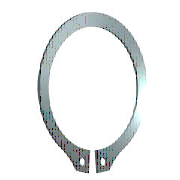
# Autodesk Inventor part: Кольцо стопорное наружное
Saved by Autodesk Inventor 2025 (Build 290162010, 162A)
## iProperties
IsCustomPart: 0
Created: 2023-01-19
Part Number: Кольцо стопорное наружное
Material: Steel, Mild
Description: American National Standard Metric Tapered Retaining Rings - Basic External Series - 3AMI
Document SubType Name: Modeling
Standard: ANSI B 27.7M
Designer: pokla
Standards Organization: ANSI
Language: en-US
Size Designation: 3AMI-17
Categories: <MemberInstance><Categories><Category DisplayName="Shaft Parts" InternalName="7f7aeb1f-a693-4053-b835-cee3144e0d98" Mnemonic="SHFT"><Category DisplayName="Circlips" InternalName="413b042a-1f46-4051-a560-0e0e417af91f" Mnemonic="CLIP"><CategoryParameter DisplayName="Thickness" InternalName="230c7f7c-2544-4c6d-b8d5-773e831b23fa" Mnemonic="thick"/><CategoryParameter DisplayName="Groove Diameter" InternalName="4054b45c-161d-4ad6-befb-f30b3855ce84" Mnemonic="grvdia"/><CategoryParameter DisplayName="Groove Width" InternalName="4dde6996-4bf1-443b-8317-d4f4fc6b9be0" Mnemonic="NB"/><CategoryParameter DisplayName="Shaft Diameter" InternalName="a433c9ab-b9eb-4798-a453-f2210a67728e" Mnemonic="shaftdia"/><Category DisplayName="External" InternalName="a9a2b132-a8be-48ab-9c3d-0c324a909558" Mnemonic="OUCLIP"><CategoryParameter DisplayName="Shaft Diameter Min." InternalName="62b77b9b-1e86-4b9a-9911-d7c0fa48fc9a" Mnemonic="shaftdiamin"/><CategoryParameter DisplayName="Outer Diameter" InternalName="a3599e7b-be7c-41b5-9a50-6dab253b0906" Mnemonic="outdia"/></Category></Category></Category><Category DisplayName="DataType" InternalName="23b78d0f-2648-40c6-8793-ca6db495c9e8" Mnemonic="DATATYPE"><CategoryParameter DisplayName="DisplayName" InternalName="05415f3d-3907-474b-a020-eb9d644f4cf3" Mnemonic="DISPLAYNAME"/><CategoryParameter DisplayName="Standard" InternalName="0c0a119c-1e12-4c84-803f-101930972f5e" Mnemonic="STANDARD"/><CategoryParameter DisplayName="Description" InternalName="13903e3d-64b1-4950-80da-f627842ea37f" Mnemonic="DESCRIPTION"/><CategoryParameter DisplayName="Designation" InternalName="2675968c-4ce5-49e0-a4f5-552d29089031" Mnemonic="DESIGNATION"/><CategoryParameter DisplayName="Default Row" InternalName="2af9ec52-faaa-4026-b378-f9fa4afca842" Mnemonic="DEFAULTROW"/><CategoryParameter DisplayName="Folder Name" InternalName="3f06958e-8713-4116-9be7-ed6184ecc97b" Mnemonic="FOLDERNAME"/><CategoryParameter DisplayName="Revision Guid" InternalName="45a75005-10b1-4dfc-8d6d-dfe629f0b93c" Mnemonic="REVISIONGUID"/><CategoryParameter DisplayName="FileName" InternalName="8b46a4cc-9585-4fed-90c3-899f57e09a73" Mnemonic="FILENAME"/><CategoryParameter DisplayName="StdsOrg" InternalName="8f5914e1-4693-403f-8ab5-d37768198c9d" Mnemonic="STDSORG"/><CategoryParameter DisplayName="Family Version" InternalName="914462f6-6e19-4b14-ba84-155b9680b1d0" Mnemonic="FAMILYREVISION"/><CategoryParameter DisplayName="Standard Revision" InternalName="91d5a463-65c2-4fde-b823-3b7fea5e8e17" Mnemonic="STANDARDREVISION"/><CategoryParameter DisplayName="Member Revision" InternalName="a65d44b9-392f-4f4f-857b-e4b3d54996fe" Mnemonic="MEMBERREVISION"/><CategoryParameter DisplayName="ClipFormat" InternalName="bc51e27b-3422-4e78-93ef-cec197ddf230" Mnemonic="CLIPFORMAT"/><CategoryParameter DisplayName="Manufacturer" InternalName="cd6c7a72-a28a-4e50-99a9-2c7f4e13e5ad" Mnemonic="MANUFACTURER"/><CategoryParameter DisplayName="InternalName" InternalName="cf1d0246-76d9-4b4a-8305-fa0409afb5c1" Mnemonic="INTERNALNAME"/><CategoryParameter DisplayName="IsMetric" InternalName="e2385c5b-1ea4-4823-96a8-8de651266ec3" Mnemonic="ISMETRIC"/><Category DisplayName="Part" InternalName="c0e0b642-3bcb-4cc8-9e80-f96d35c4afa4" Mnemonic="PART"><CategoryParameter DisplayName="Part Number" InternalName="016b6077-bfbe-49bd-92c9-d8d59c39c941" Mnemonic="PARTNUMBER"/><CategoryParameter DisplayName="Stock Number" InternalName="4dba7c1c-e26c-444e-836c-b08b433409a8" Mnemonic="STOCKNUMBER"/><CategoryParameter DisplayName="Material Key" InternalName="5c9a8adb-dd2b-4535-b97f-0a94a95fe41f" Mnemonic="MATERIALKEY"/><CategoryParameter DisplayName="Material" InternalName="818a152a-d3c3-49ca-80ee-df7d91421b8e" Mnemonic="MATERIAL"/></Category></Category><Category DisplayName="Legacy Map DA" InternalName="924fff40-ddd0-4eff-ad42-30e3774ef79e" Mnemonic="LEGACYMAPDA"><CategoryParameter DisplayName="DACookie" InternalName="316934ee-8fe1-4c7a-9c36-f2d79e1add1a" Mnemonic="DACOOKIE"/></Category></Categories><FamilyTemplate Id="A2773e"><FamilyTemplateParameters><FamilyTemplateParameter ObjectType="kUserParameterObject" ValueType="xs:double" Id="3" ObjectReferenceKey="tt"/><FamilyTemplateParameter ObjectType="kUserParameterObject" ValueType="xs:double" Id="4" ObjectReferenceKey="g1"/><FamilyTemplateParameter ObjectType="kUserParameterObject" ValueType="xs:double" Id="8" ObjectReferenceKey="Diam5"/><FamilyTemplateParameter ObjectType="kUserParameterObject" ValueType="xs:double" Id="9" ObjectReferenceKey="b"/><FamilyTemplateParameter ObjectType="kUserParameterObject" ValueType="xs:double" Id="10" ObjectReferenceKey="ParA"/><FamilyTemplateParameter ObjectType="kUserParameterObject" ValueType="xs:string" Id="117" ObjectReferenceKey="TEMPLATE"/><FamilyTemplateParameter ObjectType="kPropertyObject" ValueType="xs:string" Id="100" ObjectReferenceKey="{32853F0F-3444-11d1-9E93-0060B03C1CA6}" SubObjectId="52"/><FamilyTemplateParameter ObjectType="kPropertyObject" ValueType="xs:string" Id="105" ObjectReferenceKey="{32853F0F-3444-11d1-9E93-0060B03C1CA6}" SubObjectId="5"/><FamilyTemplateParameter ObjectType="kPartComponentDefinitionObject" ValueType="xs:string" Id="110" SubObjectId="Material"/></FamilyTemplateParameters></FamilyTemplate><CategoryParameterMap><ParamToTemplateMap><ParamToTemplate CategoryParameter="//CategoryParameter[@InternalName='05415f3d-3907-474b-a020-eb9d644f4cf3']" ConstantValue="ANSI B 27.7M"/><ParamToTemplate CategoryParameter="//CategoryParameter[@InternalName='cf1d0246-76d9-4b4a-8305-fa0409afb5c1']" ConstantValue="84A47C50-19B2-4694-A97F-23806F30E450"/><ParamToTemplate CategoryParameter="//CategoryParameter[@InternalName='3f06958e-8713-4116-9be7-ed6184ecc97b']" ConstantValue="ANSI B 27.7M(2)"/><ParamToTemplate CategoryParameter="//CategoryParameter[@InternalName='914462f6-6e19-4b14-ba84-155b9680b1d0']" ConstantValue="10"/><ParamToTemplate CategoryParameter="//CategoryParameter[@InternalName='bc51e27b-3422-4e78-93ef-cec197ddf230']" ConstantValue="CF_INVENTOR.STDPARTS"/><ParamToTemplate CategoryParameter="//CategoryParameter[@InternalName='e2385c5b-1ea4-4823-96a8-8de651266ec3']" ConstantValue="true"/><ParamToTemplate CategoryParameter="//CategoryParameter[@InternalName='13903e3d-64b1-4950-80da-f627842ea37f']" ConstantValue="American National Standard Metric Tapered Retaining Rings - Basic External Series - 3AMI"/><ParamToTemplate CategoryParameter="//CategoryParameter[@InternalName='8f5914e1-4693-403f-8ab5-d37768198c9d']" ConstantValue="ANSI"/><ParamToTemplate CategoryParameter="//CategoryParameter[@InternalName='0c0a119c-1e12-4c84-803f-101930972f5e']" ConstantValue="ANSI B 27.7M"/><ParamToTemplate CategoryParameter="//CategoryParameter[@InternalName='cd6c7a72-a28a-4e50-99a9-2c7f4e13e5ad']" TemplateParameter="104"/><ParamToTemplate CategoryParameter="//CategoryParameter[@InternalName='91d5a463-65c2-4fde-b823-3b7fea5e8e17']" TemplateParameter="103"/><ParamToTemplate CategoryParameter="//CategoryParameter[@InternalName='45a75005-10b1-4dfc-8d6d-dfe629f0b93c']" ConstantValue="d6c6cd7d-6663-4866-9fff-0a208e8d6214"/><ParamToTemplate CategoryParameter="//CategoryParameter[@InternalName='2af9ec52-faaa-4026-b378-f9fa4afca842']" ConstantValue="10"/><ParamToTemplate CategoryParameter="//CategoryParameter[@InternalName='8b46a4cc-9585-4fed-90c3-899f57e09a73']" ConstantValue="ANSI B 27.7M - 3AMI-17"/><ParamToTemplate CategoryParameter="//CategoryParameter[@InternalName='a65d44b9-392f-4f4f-857b-e4b3d54996fe']" ConstantValue="E8632F14-C031-4BBE-B420-CE7F4CDB762D"/><ParamToTemplate CategoryParameter="//CategoryParameter[@InternalName='a433c9ab-b9eb-4798-a453-f2210a67728e']" ConstantValue="17"/><ParamToTemplate CategoryParameter="//CategoryParameter[@InternalName='230c7f7c-2544-4c6d-b8d5-773e831b23fa']" ConstantValue="0,9"/><ParamToTemplate CategoryParameter="//CategoryParameter[@InternalName='4054b45c-161d-4ad6-befb-f30b3855ce84']" ConstantValue="15,75"/><ParamToTemplate CategoryParameter="//CategoryParameter[@InternalName='4dde6996-4bf1-443b-8317-d4f4fc6b9be0']" ConstantValue="1"/><ParamToTemplate CategoryParameter="//CategoryParameter[@InternalName='316934ee-8fe1-4c7a-9c36-f2d79e1add1a']" ConstantValue="*ANS~A2773AMI~3AMI-17*"/><ParamToTemplate CategoryParameter="//CategoryParameter[@InternalName='2675968c-4ce5-49e0-a4f5-552d29089031']" TemplateParameter="100"/><ParamToTemplate CategoryParameter="//CategoryParameter[@InternalName='818a152a-d3c3-49ca-80ee-df7d91421b8e']" TemplateParameter="110"/><ParamToTemplate CategoryParameter="//CategoryParameter[@InternalName='016b6077-bfbe-49bd-92c9-d8d59c39c941']" TemplateParameter="105"/></ParamToTemplateMap></CategoryParameterMap></MemberInstance>
Density: 7.85 g/cm^3
Appearance: Semi-Polished
Stock Number: Кольцо стопорное наружное 17мм
Author: pokla
Autodesk Inventor part; units mm, degrees
note: some values were not read from the file. Left out: dimensions or parameters whose unit could not be read.
ref_plane "YZ Plane" through (0, 0, 0) normal (1, 0, 0) x (0, 1, 0)
ref_plane "XZ Plane" through (0, 0, 0) normal (0, 1, 0) x (-1, 0, 0)
ref_plane "XY Plane" through (0, 0, 0) normal (0, 0, 1) x (1, 0, 0)
sketch "Sketch2" plane through (0, 0, 0) normal (0, 0, 1) x (1, 0, 0)
  line L0 (-0.6333, -11.3234) -> (-3.6933, -11.3234)
  line L1 (-0.6333, -7.5234) -> (-0.6333, -11.3234)
  arc A0 (0.6333, -7.5234) -> (-0.6333, -7.5234) centre (0, 0) ccw
  arc A1 (6.3372, -5.7408) -> (-6.3372, -5.7408) centre (0, 0.7667) ccw
  line L2 (0, -19.4467) -> (0, 17.2703) projected
  line L3 (0.6333, -11.3234) -> (3.6933, -11.3234)
  line L4 (0.6333, -7.5234) -> (0.6333, -11.3234)
  arc A2 (-3.6933, -11.3234) -> (-6.3372, -5.7408) centre (-12.514, -12.0834) ccw
  arc A3 (6.3372, -5.7408) -> (3.6933, -11.3234) centre (12.514, -12.0834) ccw
  dimension "d15" = 0.7667
  dimension "d28" = 15.1
  dimension "d32" = 2.3
  dimension "d34" = 3.8
  dimension "d35" = 1.2667
  dimension "d48" = 3.06
  dimension "d49" = 0.76
  constraints: 9 point on circle, 9 symmetric about line, 8 end point, 4 centre point, 1 coincident, 1 horizontal, 1 point on line, 1 tangent, 1 vertical, 3 other
  measures "d15" distance of A1.centre A0.centre
  measures "d28" diameter of A0
  measures "d34" distance of L1.start L0.start
  measures "d35" distance between parallel lines of L4 L1
  measures "d48" distance of L0.start L0.end
  measures "d49" distance from line of A2.centre L0
extrude "Extrusion1" add sketch "Sketch2" against normal blind 0.9
sketch "Sketch3" plane through (0, 0, 0) normal (0, 0, 1) x (1, 0, 0)
  circle A0 centre (-2.2483, -9.4234) radius 0.85
  line L0 (-0.6333, -11.3234) -> (-3.6933, -11.3234) projected
  line L1 (0.6333, -11.3234) -> (0.6333, -7.5234) projected
  line L2 (3.6933, -11.3234) -> (0.6333, -11.3234) projected
  line L3 (0, -14.2014) -> (0, -8.6014) projected
  circle A1 centre (2.2483, -9.4234) radius 0.85
  dimension "d36" = 1.7
  dimension "d37" = 1.9
  dimension "d47" = 4.4967
  constraints: 2 centre point, 1 symmetric about line, 1 other
  measures "d36" diameter of A0
  measures "d37" distance from line of L0 A0.centre
  measures "d47" diameter of A0.centre L3
extrude "Extrusion2" cut sketch "Sketch3" against normal through all
equation "\"d15\" = 0.333333 * b"
equation "\"d28\" = g1"
equation "\"d32\" = b"
equation "\"d34\" = ParA"
equation "\"d35\" = 0.333333 * ParA"
equation "\"d48\" = 1.8 * Diam5"
equation "\"d49\" = 0.2 * ParA"
equation "\"d16\" = tt"
equation "\"d36\" = Diam5"
equation "\"d37\" = 0.5 * ParA"
equation "\"d47\" = 0.333333 * ParA + 1.9 * Diam5"
equation "\"g1\" = 15.1"
equation "\"ParA\" = 3.8"
equation "\"tt\" = 0.9"
equation "\"Diam5\" = 1.7"
equation "\"TEMPLATE\" = 1.2345"
body "Solid1"
